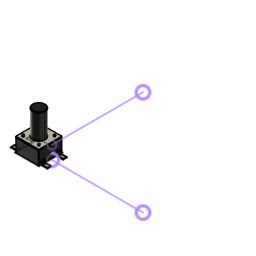
K2-1109SP-A4SA-04 (Autodesk Fusion 360 design; units mm, degrees)
Autodesk Fusion 360 part; units mm, degrees
sketch "body_and_feet" plane through (0, 0, 0) normal (0, 0, 1) x (1, 0, 0)
  line L0 (-2.25, 2.25) -> (2.25, 2.25)
  line L1 (2.25, 2.25) -> (2.25, -2.25)
  line L2 (2.25, -2.25) -> (-2.25, -2.25)
  line L3 (-2.25, -2.25) -> (-2.25, 2.25)
  line L4 (20, 0) -> (2.5, 0)
  line L5 (0, 2.5) -> (0, 20)
  line L6 (2.55, 1.85) -> (3.5, 1.85)
  line L7 (3.5, 1.85) -> (3.5, 1.15)
  line L8 (3.5, 1.15) -> (2.55, 1.15)
  line L9 (2.55, 1.15) -> (2.55, 1.85)
  line L10 (2.55, -1.15) -> (3.5, -1.15)
  line L11 (3.5, -1.15) -> (3.5, -1.85)
  line L12 (3.5, -1.85) -> (2.55, -1.85)
  line L13 (2.55, -1.85) -> (2.55, -1.15)
  line L14 (-3.5, -1.15) -> (-2.55, -1.15)
  line L15 (-2.55, -1.15) -> (-2.55, -1.85)
  line L16 (-2.55, -1.85) -> (-3.5, -1.85)
  line L17 (-3.5, -1.85) -> (-3.5, -1.15)
  line L18 (-3.5, 1.85) -> (-2.55, 1.85)
  line L19 (-2.55, 1.85) -> (-2.55, 1.15)
  line L20 (-2.55, 1.15) -> (-3.5, 1.15)
  line L21 (-3.5, 1.15) -> (-3.5, 1.85)
  dimension "d1" = 2.25
  dimension "d2" = 2.25
  dimension "d3" = 2.25
  dimension "d4" = 2.25
  dimension "d5" = 0.7
  dimension "d6" = 0.7
  dimension "d7" = 0.7
  dimension "d8" = 0.7
  dimension "d9" = 1.15
  dimension "d10" = 1.15
  dimension "d11" = 2.3
  dimension "d12" = 1.15
  dimension "d13" = 1.15
  dimension "d14" = 0.3
  dimension "d15" = 0.3
  dimension "d16" = 0.3
  dimension "d17" = 0.3
  dimension "d18" = 7
  dimension "d19" = 7
  dimension "d20" = 3.5
  dimension "d21" = 3.5
  constraint horizontal L0
  constraint vertical L1
  constraint horizontal L2
  constraint vertical L3
  constraint horizontal L6
  constraint vertical L7
  constraint horizontal L8
  constraint vertical L9
  constraint horizontal L10
  constraint vertical L11
  constraint horizontal L12
  constraint vertical L13
  constraint horizontal L14
  constraint vertical L15
  constraint horizontal L16
  constraint vertical L17
  constraint horizontal L18
  constraint vertical L19
  constraint horizontal L20
  constraint vertical L21
  measures "d1" distance of L0 L4
  measures "d2" distance of L2 L4
  measures "d3" distance of L1 L5
  measures "d4" distance of L3 L5
  measures "d5" distance of L6 L8
  measures "d6" distance of L10 L12
  measures "d7" distance of L18 L20
  measures "d8" distance of L14 L16
  measures "d9" distance of L4 L8
  measures "d10" distance of L4 L10
  measures "d11" distance of L8 L10
  measures "d12" distance of L4 L20
  measures "d13" distance of L4 L14
  measures "d14" distance of L3 L19
  measures "d15" distance of L3 L15
  measures "d16" distance of L1 L9
  measures "d17" distance of L1 L13
  measures "d18" distance of L11 L17
  measures "d19" distance of L7 L21
  measures "d20" distance of L5 L11
  measures "d21" distance of L5 L7
sketch "actuator" plane through (0, 0, 0) normal (0, 0, 1) x (1, 0, 0)
  line L0 (-2.25, -2.25) -> (-2.25, 2.25) construction
  line L1 (-2.25, 2.25) -> (2.25, 2.25) construction
  line L2 (2.25, 2.25) -> (2.25, -2.25) construction
  line L3 (2.25, -2.25) -> (-2.25, -2.25) construction
  circle A0 centre (-1.5, 1.5) radius 0.2
  circle A1 centre (1.5, 1.5) radius 0.2
  circle A2 centre (-1.5, -1.5) radius 0.2
  circle A3 centre (1.5, -1.5) radius 0.2
  line L4 (20, 0) -> (2.5, 0)
  line L5 (0, 2.5) -> (0, 20)
  circle A4 centre (0, 0) radius 1.2
  dimension "d22" = 0.4
  dimension "d23" = 0.4
  dimension "d24" = 0.4
  dimension "d25" = 0.4
  dimension "d26" = 1.5
  dimension "d27" = 1.5
  dimension "d28" = 1.5
  dimension "d29" = 1.5
  dimension "d30" = 1.5
  dimension "d31" = 1.5
  dimension "d32" = 1.5
  dimension "d33" = 1.5
  dimension "d34" = 2.4
  constraint coincident A4.centre origin
  measures "d22" diameter of A0
  measures "d23" diameter of A1
  measures "d24" diameter of A2
  measures "d25" diameter of A3
  measures "d26" distance of A0.centre L4
  measures "d27" distance of A0.centre L5
  measures "d28" distance of A1.centre L5
  measures "d29" distance of A1.centre L4
  measures "d30" distance of A3.centre L4
  measures "d31" distance of A3.centre L5
  measures "d32" distance of A2.centre L4
  measures "d33" distance of A2.centre L5
  measures "d34" diameter of A4
extrude "Extrude1" add sketch "body_and_feet" along normal blind 2.5 contours L0 L1 L2 L3 makes body 1
extrude "Extrude2" add sketch "actuator" along normal blind 4.8 from surface at 2.7 separate body contours A4 makes body 2
extrude "Extrude3" add sketch "actuator" along normal blind 0.2 from surface at 2.7 separate body contours A0 | A1 | A2 | A3 makes body 3 at (-1.301, 1.4801, 2.8333) makes body 4 at (1.699, 1.4801, 2.8333) makes body 5 at (-1.301, -1.5199, 2.8333) makes body 6 at (1.699, -1.5199, 2.8333)
extrude "Extrude4" add sketch "body_and_feet" along normal blind 0.2 from surface at 2.5 separate body contours L0 L1 L2 L3 makes body 7
extrude "Extrude5" add sketch "body_and_feet" along normal blind 0.1 separate body contours L6 L7 L8 L9 | L10 L11 L12 L13 | L14 L15 L16 L17 | L18 L19 L20 L21 makes body 8 at (-3.1833, -1.3833, 0) makes body 9 at (2.8667, -1.3833, 0) makes body 10 at (-3.1833, 1.6167, 0) makes body 11 at (2.8667, 1.6167, 0)
revolve "Revolve1" add 2 faces at (-2.55, 1.6167, 0.0333) (-2.55, -1.3833, 0.0333) angle 45 about axis through (-2.55, -1.85, 0.1) along (0, -1, 0) on bodies 8 10 bodies 10 8
revolve "Revolve2" add 2 faces at (2.55, 1.3833, 0.0333) (2.55, -1.6167, 0.0333) angle 45 about axis through (2.55, -1.15, 0.1) along (0, 1, 0) on bodies 9 11 bodies 11 9
extrude "Extrude6" add 2 faces at (-2.5029, 1.6167, 0.0529) (-2.5029, -1.3833, 0.0529) along direction (0.707107, 0, 0.707107) blind 0.2 on bodies 8 10 bodies 10 8
extrude "Extrude7" add 2 faces at (2.5029, 1.3833, 0.0529) (2.5029, -1.6167, 0.0529) along direction (-0.707107, 0, 0.707107) blind 0.2 on bodies 9 11 bodies 11 9
revolve "Revolve3" add 2 faces at (-2.3614, -1.3833, 0.1943) (-2.3614, 1.6167, 0.1943) angle 45 about axis through (-2.4086, -1.15, 0.2414) along (0, -1, 0) on bodies 8 10 bodies 8 10
revolve "Revolve4" add 2 faces at (2.3614, 1.3833, 0.1943) (2.3614, -1.6167, 0.1943) angle 45 about axis through (2.4086, -1.85, 0.2414) along (0, 1, 0) on bodies 9 11 bodies 11 9
extrude "Extrude8" add 2 faces at (-2.3419, -1.3833, 0.2414) (-2.3419, 1.6167, 0.2414) along direction (0, 0, 1) blind 0.3 on bodies 8 10 bodies 8 10
extrude "Extrude9" add 2 faces at (2.3419, -1.6167, 0.2414) (2.3419, 1.3833, 0.2414) along direction (0, 0, 1) blind 0.3 on bodies 9 11 bodies 9 11
revolve "Revolve5" add 2 faces at (-2.3419, -1.3833, 0.5414) (-2.3419, 1.6167, 0.5414) angle 45 about axis through (-2.3086, -1.85, 0.5414) along (0, 1, 0) on bodies 8 10 bodies 8 10
revolve "Revolve6" add 2 faces at (2.3419, -1.6167, 0.5414) (2.3419, 1.3833, 0.5414) angle 45 about axis through (2.3086, -1.15, 0.5414) along (0, -1, 0) on bodies 9 11 bodies 9 11
extrude "Extrude10" add 2 faces at (-2.3321, -1.3833, 0.565) (-2.3321, 1.6167, 0.565) along direction (0.707107, 0, 0.707107) blind 0.2 on bodies 8 10 bodies 8 10
extrude "Extrude11" add 2 faces at (2.3321, 1.3833, 0.565) (2.3321, -1.6167, 0.565) along direction (-0.707107, 0, 0.707107) blind 0.2 on bodies 9 11 bodies 11 9
fillet "Fillet1" radius 0.1 1 edges at (-1.1188, -0.4339, 7.5) on bodies 2
fillet "Fillet2" radius 0.05 4 edges at (0, -2.25, 2.7) (-2.25, 0, 2.7) (2.25, 0, 2.7) (0, 2.25, 2.7) on bodies 7
fillet "Fillet3" radius 0.1 12 edges at (-2.25, 2.25, 1.25) (-2.25, -2.25, 1.25) (2.25, -2.25, 1.25) (2.25, 2.25, 1.25) (-2.25, 2.25, 2.575) (-2.2354, 2.2354, 2.6854) (-2.25, -2.25, 2.575) (-2.2354, -2.2354, 2.6854) (2.25, -2.25, 2.575) (2.2354, -2.2354, 2.6854) (2.25, 2.25, 2.575) (2.2354, 2.2354, 2.6854) on bodies 1 7
